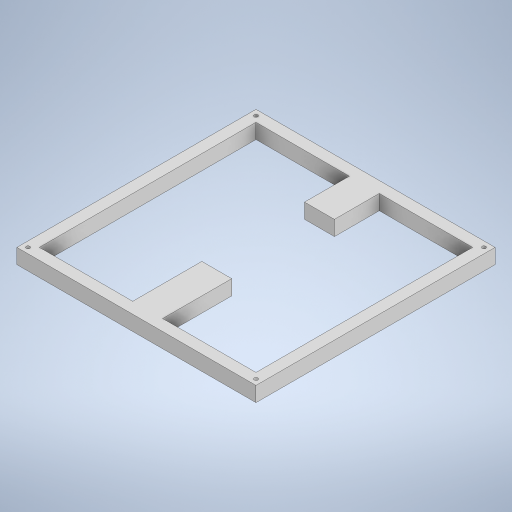
# Autodesk Inventor part: Layer 2
Saved by Autodesk Inventor 2023 (Build 270158000, 158)
## iProperties
Created: 2023-04-21
Part Number: Layer 2
Material: Generic
Document SubType Name: Modeling
Designer: byrne
Density: 1 g/cm^3
Appearance: Default
Author: byrne
Autodesk Inventor part; units mm, degrees
ref_plane "YZ Plane" through (0, 0, 0) normal (1, 0, 0) x (0, 1, 0)
ref_plane "XZ Plane" through (0, 0, 0) normal (0, 1, 0) x (-1, 0, 0)
ref_plane "XY Plane" through (0, 0, 0) normal (0, 0, 1) x (1, 0, 0)
sketch "Sketch1" plane through (0, 0, 0) normal (0, 1, 0) x (-1, 0, 0)
  line L0 (0, 0) -> (101.6, 0)
  line L1 (101.6, 0) -> (101.6, -101.6)
  line L2 (101.6, -101.6) -> (0, -101.6)
  line L3 (0, -101.6) -> (0, 0)
  line L4 (4.7625, -96.8375) -> (96.8375, -96.8375)
  line L5 (96.8375, -96.8375) -> (96.8375, -4.7625)
  line L6 (96.8375, -4.7625) -> (4.7625, -4.7625)
  line L7 (4.7625, -4.7625) -> (4.7625, -96.8375)
  line L8 (57.15, -4.7625) -> (44.45, -4.7625)
  line L9 (44.45, -4.7625) -> (44.45, -34.1313)
  line L10 (44.45, -34.1313) -> (57.15, -34.1313)
  line L11 (57.15, -34.1313) -> (57.15, -4.7625)
  line L12 (57.15, -96.8375) -> (44.45, -96.8375)
  line L13 (44.45, -96.8375) -> (44.45, -77.7875)
  line L14 (44.45, -77.7875) -> (57.15, -77.7875)
  line L15 (57.15, -77.7875) -> (57.15, -96.8375)
  line L16 (57.15, -34.1312) -> (44.45, -34.1312)
  line L17 (44.45, -34.1312) -> (44.45, -57.15) construction
  line L18 (44.45, -57.15) -> (57.15, -57.15) construction
  line L19 (57.15, -57.15) -> (57.15, -34.1312) construction
  point P0 (50.8, -50.8)
  point P1 (0, -50.8)
  point P2 (50.8, 0)
  point P3 (50.8, -4.7625)
  point P4 (50.8, -4.7625)
  point P5 (50.8, -96.8375)
  point P6 (50.8, -96.8375)
  point P7 (50.8, -34.1312)
  point P8 (50.8, -34.1313)
  point P9 (50.8, -50.8)
  point P10 (50.8, -57.15)
  dimension "d0" = 101.6
  dimension "d1" = 101.6
  dimension "d2" = 4.7625
  dimension "d13" = 12.7
  dimension "d15" = 29.3687
  dimension "d16" = 12.7
  dimension "d17" = 23.0188
  dimension "d18" = 6.35
  dimension "d33" = 19.05
  constraints: 40 end point, 10 parallel, 9 midpoint, 5 perpendicular, 4 coincident, 4 collinear, 4 horizontal, 2 vertical alignment, 1 horizontal alignment, 3 other
  measures "d0" distance of L1.end L2.end
  measures "d1" distance of L0.end L1.end
  measures "d2" distance between parallel lines of L2 L4
  measures "d13" distance of L9.end L10.end
  measures "d15" distance of L10.end L8.start
  measures "d16" distance between parallel lines of L17 L19
  measures "d17" distance between parallel lines of L18 L16
  measures "d18" distance from line of L18 point (50.8, -50.8)
  measures "d33" distance of L12.end L13.end
extrude "Extrusion1" add sketch "Sketch1" along normal blind 6.35 contours L0 L1 L2 L3 | L13 L14 L15 L4 | L6 L11 L10 L9
sketch "Sketch2" plane through (0, 6.35, 0) normal (0, 1, 0) x (1, 0, 0)
  line L0 (0, 101.6) -> (-101.6, 101.6) projected
  line L1 (-101.6, 101.6) -> (-101.6, 0) projected
  line L2 (-101.6, 0) -> (0, 0) projected
  line L3 (0, 0) -> (0, 101.6) projected
  circle A0 centre (-99.2188, 99.2188) radius 0.7938
  circle A1 centre (-99.2188, 2.3813) radius 0.7938
  circle A2 centre (-2.3813, 99.2188) radius 0.7938
  circle A3 centre (-2.3813, 2.3813) radius 0.7938
  dimension "d20" = 1.5875
  dimension "d21" = 2.3813
  dimension "d22" = 2.3813
  dimension "d25" = 96.8375
  dimension "d28" = 96.8375
  constraints: 4 centre point, 1 horizontal, 1 vertical, 6 other
  measures "d20" diameter of A0
  measures "d21" distance from line of L0 A0.centre
  measures "d22" distance from line of L1 A0.centre
  measures "d25" distance of A0.centre A1.centre
  measures "d28" distance of A0.centre A2.centre
extrude "Extrusion2" cut sketch "Sketch2" against normal blind 6.35 contours A0 | A1 | A2 | A3
sketch "Sketch3" plane through (0, 6.35, 0) normal (0, 1, 0) x (1, 0, 0)
  circle A0 centre (-99.2188, 99.2188) radius 0.7938 projected
  circle A1 centre (-99.2188, 2.3813) radius 0.7938 projected
  circle A2 centre (-2.3813, 99.2188) radius 0.7938 projected
  circle A3 centre (-2.3813, 2.3813) radius 0.7938 projected
  line L0 (0, 101.6) -> (-101.6, 101.6) projected
  line L1 (-101.6, 101.6) -> (-101.6, 0) projected
  line L2 (-101.6, 0) -> (0, 0) projected
  line L3 (0, 0) -> (0, 101.6) projected
  line L4 (-96.8375, 4.7625) -> (-96.8375, 96.8375) projected
  line L5 (-96.8375, 96.8375) -> (-57.15, 96.8375) projected
  line L6 (-57.15, 96.8375) -> (-57.15, 77.7875) projected
  line L7 (-57.15, 77.7875) -> (-44.45, 77.7875) projected
  line L8 (-44.45, 77.7875) -> (-44.45, 96.8375) projected
  line L9 (-44.45, 96.8375) -> (-4.7625, 96.8375) projected
  line L10 (-4.7625, 96.8375) -> (-4.7625, 4.7625) projected
  line L11 (-4.7625, 4.7625) -> (-44.45, 4.7625) projected
  line L12 (-44.45, 4.7625) -> (-44.45, 34.1313) projected
  line L13 (-44.45, 34.1313) -> (-57.15, 34.1313) projected
  line L14 (-57.15, 34.1313) -> (-57.15, 4.7625) projected
  line L15 (-57.15, 4.7625) -> (-96.8375, 4.7625) projected
body "Solid1"
